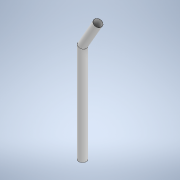
# Autodesk Inventor part: feedthroughpip2
Saved by Autodesk Inventor 2020 (Build 240168000, 168)
## iProperties
Created: 2019-07-29
Part Number: feedthroughpip2
Material: Generic
Document SubType Name: Modeling
Designer: ColinP
Density: 1 g/cm^3
Appearance: Default
Author: ColinP
Autodesk Inventor part; units mm, degrees
ref_plane "YZ Plane" through (0, 0, 0) normal (1, 0, 0) x (0, 1, 0)
ref_plane "XZ Plane" through (0, 0, 0) normal (0, 1, 0) x (-1, 0, 0)
ref_plane "XY Plane" through (0, 0, 0) normal (0, 0, 1) x (1, 0, 0)
sketch "Sketch1" plane through (0, 0, 0) normal (0, 1, 0) x (-1, 0, 0)
  circle A0 centre (0, 0) radius 3.175
  circle A1 centre (0, 0) radius 3.048
  dimension "d0" = 6.35
  dimension "d1" = 6.096
  constraints: 2 centre point, 2 coincident
  measures "d0" diameter of A0
  measures "d1" diameter of A1
sketch "Sketch2" plane through (0, 0, 0) normal (0, 0, 1) x (1, 0, 0)
  line L0 (0, 0) -> (0, 81.28)
  line L1 (0, 81.28) -> (0, 73.4379)
  line L2 (0, 81.28) -> (12.6562, 103.3023)
  line L3 (0, 81.28) -> (25.4, 81.28) construction
  dimension "d2" = 81.28
  dimension "d3" = 25.4
  dimension "d4" = 60.114
  constraints: 8 end point, 1 equal length, 1 horizontal, 1 point on line, 1 vertical
  measures "d2" distance of L0.start L0.end
  measures "d3" distance of L0.end L2.end
  measures "d4" angle of L3 L2
sweep "Sweep1" add profiles "Sketch1" path "Sketch2" path curves L0 L2
body "Solid1"
